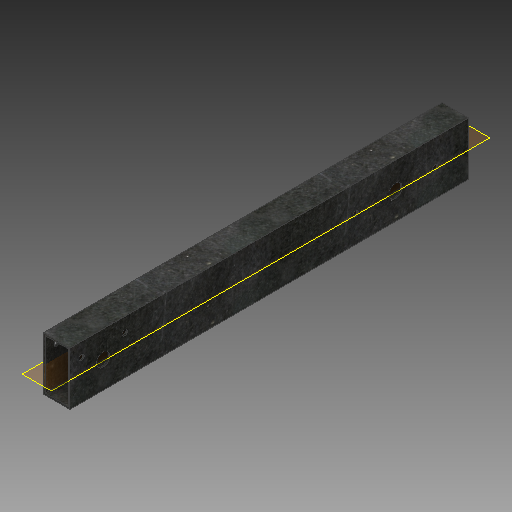
# Autodesk Inventor part: Steel 4130 1x2in. Tubing, t=.065in.,L=15in.
Saved by Autodesk Inventor 2019 (Build 230136000, 136)
## iProperties
Created: 2018-10-28
Part Number: Steel 4130 1x2in. Tubing, t=.065in.,L=15in.
Material: Steel
Document SubType Name: Modeling
Designer: Alex Barnett
Density: 7.85 g/cm^3
Appearance: Plate
Author: Alex Barnett
Autodesk Inventor part; units mm, degrees
ref_plane "YZ Plane" through (0, 0, 0) normal (1, 0, 0) x (0, 1, 0)
ref_plane "XY Plane" through (0, 0, 0) normal (0, 0, 1) x (1, 0, 0)
sketch "Sketch1" plane through (0, 0, 0) normal (0, 0, 1) x (1, 0, 0)
  line L0 (-12.7, -25.4) -> (12.7, -25.4)
  line L1 (12.7, -25.4) -> (12.7, 25.4)
  line L2 (12.7, 25.4) -> (-12.7, 25.4)
  line L3 (-12.7, 25.4) -> (-12.7, -25.4)
  line L4 (-12.7, -25.4) -> (12.7, 25.4) construction
  line L5 (12.7, -25.4) -> (-12.7, 25.4) construction
  line L6 (-11.049, -23.749) -> (11.049, -23.749)
  line L7 (11.049, -23.749) -> (11.049, 23.749)
  line L8 (11.049, 23.749) -> (-11.049, 23.749)
  line L9 (-11.049, 23.749) -> (-11.049, -23.749)
  line L10 (-11.049, -23.749) -> (11.049, 23.749) construction
  line L11 (11.049, -23.749) -> (-11.049, 23.749) construction
  point P0 (0, 0)
  dimension "d0" = 25.4
  dimension "d1" = 50.8
  dimension "d4" = 22.098
  dimension "d5" = 47.498
  constraints: 24 end point, 4 midpoint, 4 parallel, 2 horizontal, 2 perpendicular
  measures "d0" distance of L2.end L1.end
  measures "d1" distance of L1.end L0.end
  measures "d4" distance of L8.end L7.end
  measures "d5" distance of L7.end L6.end
extrude "Extrusion2" add sketch "Sketch1" along normal mid plane 381
sketch "Sketch2" plane through (12.7, -25.4, 190.5) normal (1, 0, 0) x (0, 0, -1)
  line L0 (381, 50.8) -> (0, 50.8) projected
  line L1 (0, 0) -> (0, 50.8) projected
  line L2 (381, 0) -> (0, 0) projected
  line L3 (381, 50.8) -> (381, 0) projected
  line L4 (31.75, 25.4) -> (-38.0984, 65.727) construction
  line L5 (31.75, 25.4) -> (112.404, 25.4) construction
  line L6 (31.75, 25.4) -> (122.705, 77.9129) construction
  line L7 (31.75, 25.4) -> (136.7757, 25.4) construction
  line L8 (31.75, 25.4) -> (31.75, -25.6203) construction
  circle A0 centre (31.75, 25.4) radius 23.8125 construction
  point P0 (190.5, 25.4)
  point P1 (11.1278, 37.3063)
  point P2 (52.3722, 37.3063)
  dimension "d8" = 31.75
  dimension "d9" = 25.4
  dimension "d10" = 150
  dimension "d11" = 30
  dimension "d12" = 47.625
  dimension "d20" = 0
  dimension "d21" = 0
  constraints: 10 end point, 2 equal length, 2 horizontal, 2 point on circle, 2 point on line, 1 centre point, 1 vertical
  measures "d8" distance from line of L1 L4.start
  measures "d9" distance from line of L0 L4.start
  measures "d10" angle of L5 L4
  measures "d11" angle of L7 L6
  measures "d12" diameter of A0
  measures "d20" distance of L4.start A0.centre
  measures "d21" distance of L4.start A0.centre
hole "Hole1" at (12.7, 11.9063, 179.3722) at (12.7, 11.9063, 138.1278) direction (-1, 0, 0) diameter 5.08 end through all
sketch "Sketch3" plane through (12.7, -25.4, 190.5) normal (1, 0, 0) x (0, 0, -1)
  circle A0 centre (11.1278, 37.3063) radius 2.54 projected
  circle A1 centre (52.3722, 37.3063) radius 2.54 projected
  line L0 (381, 50.8) -> (0, 50.8) projected
  line L1 (0, 0) -> (0, 50.8) projected
  line L2 (381, 0) -> (0, 0) projected
  line L3 (381, 50.8) -> (381, 0) projected
  circle A2 centre (31.75, 25.4) radius 6.35
  point P0 (190.5, 25.4)
  dimension "d22" = 12.7
  dimension "d23" = 31.75
  dimension "d24" = 25.4
  constraints: 1 centre point
  measures "d22" diameter of A2
  measures "d23" distance from line of L1 A2.centre
  measures "d24" distance from line of L0 A2.centre
hole "Hole2" at (12.7, 0, 158.75) direction (-1, 0, 0) diameter 12.7 end through all
sketch "Sketch4" plane through (12.7, -25.4, 190.5) normal (1, 0, 0) x (0, 0, -1)
  circle A0 centre (31.75, 25.4) radius 6.35 projected
  circle A1 centre (11.1278, 37.3063) radius 2.54 projected
  circle A2 centre (52.3722, 37.3063) radius 2.54 projected
  line L0 (381, 50.8) -> (0, 50.8) projected
  line L1 (0, 0) -> (0, 50.8) projected
  line L2 (381, 0) -> (0, 0) projected
  line L3 (381, 50.8) -> (381, 0) projected
  point P0 (190.5, 25.4)
  point P1 (311.15, 25.4)
  dimension "d32" = 69.85
  dimension "d33" = 25.4
  measures "d32" distance from line of L3 point (311.15, 25.4)
  measures "d33" distance from line of L0 point (311.15, 25.4)
hole "Hole3" at (12.7, 0, -120.65) direction (-1, 0, 0) diameter 12.7 end through all
sketch "Sketch5" plane through (12.7, -25.4, 190.5) normal (1, 0, 0) x (0, 0, -1)
  circle A0 centre (311.15, 25.4) radius 6.35 projected
  circle A1 centre (31.75, 25.4) radius 6.35 projected
  circle A2 centre (11.1278, 37.3063) radius 2.54 projected
  circle A3 centre (52.3722, 37.3063) radius 2.54 projected
  line L0 (381, 50.8) -> (0, 50.8) projected
  line L1 (0, 0) -> (0, 50.8) projected
  line L2 (381, 0) -> (0, 0) projected
  line L3 (381, 50.8) -> (381, 0) projected
  point P0 (190.5, 25.4)
  point P1 (349.25, 25.4)
  point P2 (273.05, 25.4)
  dimension "d41" = 76.2
  dimension "d42" = 38.1
  measures "d41" distance of point (273.05, 25.4) point (349.25, 25.4)
  measures "d42" distance of A0.centre point (349.25, 25.4)
hole "Hole4" at (12.7, 0, -158.75) at (12.7, 0, -82.55) direction (-1, 0, 0) diameter 5.08 end through all
body "Solid2"
